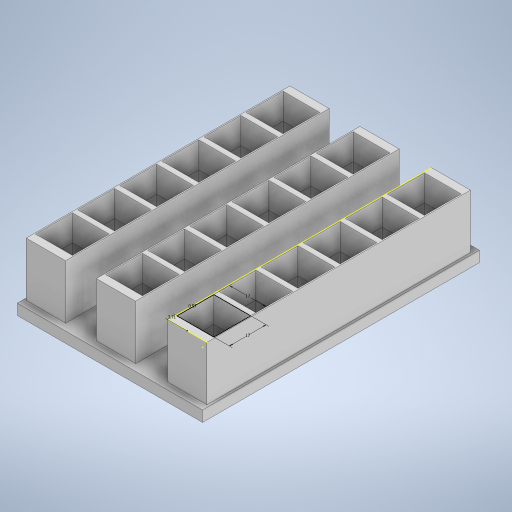
# Autodesk Inventor part: cuvettestorage3_6x3
Saved by Autodesk Inventor 2023 (Build 270158000, 158)
## iProperties
Created: 2024-07-02
Part Number: cuvettestorage3_6x3
Material: Generic
Document SubType Name: Modeling
Designer: storm
Density: 1 g/cm^3
Appearance: Default
Author: storm
Autodesk Inventor part; units mm, degrees
ref_plane "YZ Plane" through (0, 0, 0) normal (1, 0, 0) x (0, 1, 0)
ref_plane "XZ Plane" through (0, 0, 0) normal (0, 1, 0) x (-1, 0, 0)
ref_plane "XY Plane" through (0, 0, 0) normal (0, 0, 1) x (1, 0, 0)
sketch "Sketch1" plane through (0, 0, 0) normal (0, 1, 0) x (-1, 0, 0)
  line L0 (0, 0) -> (85.5, 0)
  line L1 (85.5, 0) -> (85.5, -127.8)
  line L2 (85.5, -127.8) -> (0, -127.8)
  line L3 (0, -127.8) -> (0, 0)
  dimension "d0" = 127.8
  dimension "d1" = 85.5
  constraints: 8 end point, 2 parallel, 1 horizontal, 1 perpendicular
  measures "d0" distance of L0.end L1.end
  measures "d1" distance between parallel lines of L3 L1
extrude "Extrusion1" add sketch "Sketch1" along normal blind 5
sketch "Sketch2" plane through (0, 5, 0) normal (0, 1, 0) x (1, 0, 0)
  line L0 (-84.43, 3.05) -> (-66.3, 3.05)
  line L1 (-66.3, 3.05) -> (-66.3, 124.74)
  line L2 (-66.3, 124.74) -> (-84.43, 124.74)
  line L3 (-84.43, 124.74) -> (-84.43, 3.05)
  line L4 (-52.08, 3.05) -> (-33.95, 3.05)
  line L5 (-33.95, 3.05) -> (-33.95, 124.74)
  line L6 (-33.95, 124.74) -> (-52.08, 124.74)
  line L7 (-52.08, 124.74) -> (-52.08, 3.05)
  line L8 (-19.18, 3.05) -> (-1.05, 3.05)
  line L9 (-1.05, 3.05) -> (-1.05, 124.74)
  line L10 (-1.05, 124.74) -> (-19.18, 124.74)
  line L11 (-19.18, 124.74) -> (-19.18, 3.05)
  line L12 (0, 0) -> (0, 127.8) projected
  line L13 (-85.5, 0) -> (0, 0) projected
  point P0 (-10.115, 124.74)
  point P1 (-10.115, 3.05)
  dimension "d4" = 18.13
  dimension "d5" = 121.69
  dimension "d6" = 1.05
  dimension "d7" = 3.05
  dimension "d8" = 14.77
  dimension "d9" = 18.13
  dimension "d10" = 14.22
  dimension "d11" = 18.13
  constraints: 24 end point, 6 parallel, 4 point on line, 3 horizontal, 3 perpendicular, 2 midpoint
  measures "d4" distance between parallel lines of L9 L11
  measures "d5" distance of point (-10.115, 124.74) point (-10.115, 3.05)
  measures "d6" distance between parallel lines of L12 L9
  measures "d7" distance between parallel lines of L13 L8
  measures "d8" distance between parallel lines of L11 L5
  measures "d9" distance between parallel lines of L5 L7
  measures "d10" distance between parallel lines of L7 L1
  measures "d11" distance between parallel lines of L1 L3
extrude "Extrusion2" add sketch "Sketch2" along normal blind 25
sketch "Sketch3" plane through (0, 30, 0) normal (0, 1, 0) x (1, 0, 0)
  line L0 (-19.18, 124.74) -> (-19.18, 3.05) projected
  line L1 (-1.05, 3.05) -> (-1.05, 124.74) projected
  line L2 (-19.18, 3.05) -> (-1.05, 3.05) projected
  line L3 (-16.615, 28.214) -> (-3.615, 28.214)
  line L4 (-3.615, 28.214) -> (-3.615, 41.214)
  line L5 (-3.615, 41.214) -> (-16.615, 41.214)
  line L6 (-16.615, 41.214) -> (-16.615, 28.214)
  line L7 (-16.615, 47.668) -> (-3.615, 47.668)
  line L8 (-3.615, 47.668) -> (-3.615, 60.668)
  line L9 (-3.615, 60.668) -> (-16.615, 60.668)
  line L10 (-16.615, 60.668) -> (-16.615, 47.668)
  line L11 (-16.615, 67.122) -> (-3.615, 67.122)
  line L12 (-3.615, 67.122) -> (-3.615, 80.122)
  line L13 (-3.615, 80.122) -> (-16.615, 80.122)
  line L14 (-16.615, 80.122) -> (-16.615, 67.122)
  line L15 (-16.615, 86.576) -> (-3.615, 86.576)
  line L16 (-3.615, 86.576) -> (-3.615, 99.576)
  line L17 (-3.615, 99.576) -> (-16.615, 99.576)
  line L18 (-16.615, 99.576) -> (-16.615, 86.576)
  line L19 (-16.615, 106.03) -> (-3.615, 106.03)
  line L20 (-3.615, 106.03) -> (-3.615, 119.03)
  line L21 (-3.615, 119.03) -> (-16.615, 119.03)
  line L22 (-16.615, 119.03) -> (-16.615, 106.03)
  line L23 (-1.05, 124.74) -> (-19.18, 124.74) projected
  line L24 (-52.08, 124.74) -> (-52.08, 3.05) projected
  line L25 (-33.95, 3.05) -> (-33.95, 124.74) projected
  line L26 (-52.08, 3.05) -> (-33.95, 3.05) projected
  line L27 (-84.43, 124.74) -> (-84.43, 3.05) projected
  line L28 (-66.3, 3.05) -> (-66.3, 124.74) projected
  line L29 (-84.43, 3.05) -> (-66.3, 3.05) projected
  line L30 (-16.615, 8.76) -> (-3.615, 8.76)
  line L31 (-3.615, 8.76) -> (-3.615, 21.76)
  line L32 (-3.615, 21.76) -> (-16.615, 21.76)
  line L33 (-16.615, 21.76) -> (-16.615, 8.76)
  line L34 (-33.95, 124.74) -> (-52.08, 124.74) projected
  line L35 (-49.515, 8.76) -> (-36.515, 8.76)
  line L36 (-36.515, 8.76) -> (-36.515, 21.76)
  line L37 (-36.515, 21.76) -> (-49.515, 21.76)
  line L38 (-49.515, 21.76) -> (-49.515, 8.76)
  line L39 (-49.515, 28.214) -> (-36.515, 28.214)
  line L40 (-36.515, 28.214) -> (-36.515, 41.214)
  line L41 (-36.515, 41.214) -> (-49.515, 41.214)
  line L42 (-49.515, 41.214) -> (-49.515, 28.214)
  line L43 (-49.515, 47.668) -> (-36.515, 47.668)
  line L44 (-36.515, 47.668) -> (-36.515, 60.668)
  line L45 (-36.515, 60.668) -> (-49.515, 60.668)
  line L46 (-49.515, 60.668) -> (-49.515, 47.668)
  line L47 (-49.515, 67.122) -> (-36.515, 67.122)
  line L48 (-36.515, 67.122) -> (-36.515, 80.122)
  line L49 (-36.515, 80.122) -> (-49.515, 80.122)
  line L50 (-49.515, 80.122) -> (-49.515, 67.122)
  line L51 (-49.515, 86.576) -> (-36.515, 86.576)
  line L52 (-36.515, 86.576) -> (-36.515, 99.576)
  line L53 (-36.515, 99.576) -> (-49.515, 99.576)
  line L54 (-49.515, 99.576) -> (-49.515, 86.576)
  line L55 (-49.515, 106.03) -> (-36.515, 106.03)
  line L56 (-36.515, 106.03) -> (-36.515, 119.03)
  line L57 (-36.515, 119.03) -> (-49.515, 119.03)
  line L58 (-49.515, 119.03) -> (-49.515, 106.03)
  line L59 (-81.865, 8.76) -> (-68.865, 8.76)
  line L60 (-68.865, 8.76) -> (-68.865, 21.76)
  line L61 (-68.865, 21.76) -> (-81.865, 21.76)
  line L62 (-81.865, 21.76) -> (-81.865, 8.76)
  line L63 (-81.865, 28.214) -> (-68.865, 28.214)
  line L64 (-68.865, 28.214) -> (-68.865, 41.214)
  line L65 (-68.865, 41.214) -> (-81.865, 41.214)
  line L66 (-81.865, 41.214) -> (-81.865, 28.214)
  line L67 (-81.865, 47.668) -> (-68.865, 47.668)
  line L68 (-68.865, 47.668) -> (-68.865, 60.668)
  line L69 (-68.865, 60.668) -> (-81.865, 60.668)
  line L70 (-81.865, 60.668) -> (-81.865, 47.668)
  line L71 (-81.865, 67.122) -> (-68.865, 67.122)
  line L72 (-68.865, 67.122) -> (-68.865, 80.122)
  line L73 (-68.865, 80.122) -> (-81.865, 80.122)
  line L74 (-81.865, 80.122) -> (-81.865, 67.122)
  line L75 (-81.865, 86.576) -> (-68.865, 86.576)
  line L76 (-68.865, 86.576) -> (-68.865, 99.576)
  line L77 (-68.865, 99.576) -> (-81.865, 99.576)
  line L78 (-81.865, 99.576) -> (-81.865, 86.576)
  line L79 (-81.865, 106.03) -> (-68.865, 106.03)
  line L80 (-68.865, 106.03) -> (-68.865, 119.03)
  line L81 (-68.865, 119.03) -> (-81.865, 119.03)
  line L82 (-81.865, 119.03) -> (-81.865, 106.03)
  line L83 (-66.3, 124.74) -> (-84.43, 124.74) projected
  point P0 (0, 0)
  point P1 (-16.615, 13.26)
  point P2 (-3.615, 13.26)
  point P3 (-10.115, 60.668)
  point P4 (-10.115, 47.668)
  point P5 (-3.615, 54.168)
  point P6 (-16.615, 54.168)
  point P7 (-16.615, 73.622)
  point P8 (-3.615, 93.076)
  point P9 (-16.615, 93.076)
  point P10 (-3.615, 112.53)
  point P11 (-16.615, 112.53)
  point P12 (-3.615, 34.714)
  point P13 (-1.05, 63.895)
  point P14 (-10.115, 80.122)
  point P15 (-10.115, 41.214)
  point P16 (-10.115, 28.214)
  point P17 (-43.015, 3.05)
  point P18 (-75.365, 3.05)
  point P19 (-10.115, 8.76)
  point P20 (-10.115, 3.05)
  point P21 (-43.015, 124.74)
  point P22 (-43.015, 8.76)
  point P23 (-49.515, 15.26)
  point P24 (-75.365, 21.76)
  point P25 (-75.365, 67.122)
  point P26 (-75.365, 60.668)
  point P27 (-75.365, 106.03)
  point P28 (-75.365, 99.576)
  point P29 (-75.365, 124.74)
  point P30 (-68.865, 15.26)
  dimension "d19" = 13
  dimension "d20" = 13
  dimension "d21" = 13
  dimension "d22" = 13
  dimension "d23" = 13
  dimension "d24" = 13
  dimension "d25" = 13
  dimension "d26" = 13
  dimension "d27" = 13
  dimension "d28" = 13
  dimension "d29" = 5.71
  dimension "d33" = 2.565
  dimension "d34" = 2.565
  dimension "d35" = 2.565
  dimension "d36" = 2.565
  dimension "d37" = 2.565
  dimension "d38" = 2.565
  dimension "d39" = 2.565
  dimension "d40" = 121.69
  dimension "d41" = 6.454
  dimension "d42" = 6.454
  dimension "d43" = 6.454
  dimension "d44" = 6.454
  dimension "d67" = 6.454
  dimension "d68" = 5.71
  dimension "d78" = 13
  dimension "d79" = 13
  dimension "d80" = 5.71
  dimension "d81" = 2.565
  dimension "d82" = 2.565
  dimension "d83" = 6.454
  dimension "d84" = 6.454
  dimension "d85" = 6.454
  dimension "d86" = 6.454
  dimension "d87" = 6.454
  dimension "d88" = 13
  dimension "d89" = 5.71
  dimension "d90" = 6.454
  dimension "d91" = 6.454
  dimension "d92" = 6.454
  dimension "d93" = 6.454
  dimension "d94" = 6.454
  dimension "d95" = 5.71
  dimension "d96" = 2.565
  constraints: 144 end point, 36 parallel, 28 midpoint, 24 point on line, 18 horizontal, 18 perpendicular
  measures "d19" distance of L4.end L3.end
  measures "d20" distance between parallel lines of L4 L6
  measures "d21" distance of point (-10.115, 60.668) point (-10.115, 47.668)
  measures "d22" distance of point (-3.615, 54.168) point (-16.615, 54.168)
  measures "d23" distance from line of L12 point (-16.615, 73.622)
  measures "d24" distance between parallel lines of L13 L11
  measures "d25" distance of point (-3.615, 93.076) point (-16.615, 93.076)
  measures "d26" distance between parallel lines of L17 L15
  measures "d27" distance of point (-3.615, 112.53) point (-16.615, 112.53)
  measures "d28" distance between parallel lines of L21 L19
  measures "d29" distance between parallel lines of L23 L21
  measures "d33" distance between parallel lines of L0 L6
  measures "d34" distance from line of L1 point (-3.615, 34.714)
  measures "d35" distance between parallel lines of L0 L10
  measures "d36" distance between parallel lines of L0 L14
  measures "d37" distance from line of point (-1.05, 63.895) L12
  measures "d38" distance between parallel lines of L0 L18
  measures "d39" distance between parallel lines of L0 L22
  measures "d40" distance between parallel lines of L23 L2
  measures "d41" distance between parallel lines of L19 L17
  measures "d42" distance from line of point (-10.115, 80.122) L15
  measures "d43" distance between parallel lines of L9 L11
  measures "d44" distance from line of point (-10.115, 41.214) L7
  measures "d67" distance between parallel lines of L3 L32
  measures "d68" distance of point (-10.115, 8.76) point (-10.115, 3.05)
  measures "d78" distance of L37.end L36.end
  measures "d79" distance of L36.end L35.end
  measures "d80" distance from line of L26 point (-43.015, 8.76)
  measures "d81" distance between parallel lines of L25 L36
  measures "d82" distance from line of L24 point (-49.515, 15.26)
  measures "d83" distance between parallel lines of L39 L37
  measures "d84" distance between parallel lines of L43 L41
  measures "d85" distance between parallel lines of L47 L45
  measures "d86" distance between parallel lines of L51 L49
  measures "d87" distance between parallel lines of L55 L53
  measures "d88" distance of L61.end L60.end
  measures "d89" distance between parallel lines of L59 L29
  measures "d90" distance from line of L63 point (-75.365, 21.76)
  measures "d91" distance between parallel lines of L67 L65
  measures "d92" distance of point (-75.365, 67.122) point (-75.365, 60.668)
  measures "d93" distance between parallel lines of L75 L73
  measures "d94" distance of point (-75.365, 106.03) point (-75.365, 99.576)
  measures "d95" distance from line of L81 point (-75.365, 124.74)
  measures "d96" distance from line of L28 point (-68.865, 15.26)
extrude "Extrusion3" cut sketch "Sketch3" against normal blind 20 contours L6 L5 L4 L3 | L10 L9 L8 L7 | L14 L13 L12 L11 | L18 L17 L16 L15 | L22 L21 L20 L19
sketch "Sketch4" plane through (0, 30, 0) normal (0, 1, 0) x (1, 0, 0)
  line L0 (-16.615, 21.76) -> (-3.615, 21.76)
  line L1 (-3.615, 21.76) -> (-3.615, 8.76)
  line L2 (-3.615, 8.76) -> (-16.615, 8.76)
  line L3 (-16.615, 8.76) -> (-16.615, 21.76)
  line L4 (-19.18, 124.74) -> (-19.18, 3.05) projected
  line L5 (-1.05, 3.05) -> (-1.05, 124.74) projected
  line L6 (-19.18, 3.05) -> (-1.05, 3.05) projected
  point P0 (0, 0)
  point P1 (-16.615, 15.26)
  point P2 (-3.615, 15.26)
  point P3 (-10.115, 3.05)
  point P4 (-10.115, 8.76)
  dimension "d56" = 13
  dimension "d57" = 13
  dimension "d58" = 2.565
  dimension "d59" = 2.565
  dimension "d60" = 5.71
  constraints: 8 end point, 4 midpoint, 2 parallel, 1 horizontal, 1 perpendicular
  measures "d56" distance of L1.end L2.end
  measures "d57" distance of L0.end L1.end
  measures "d58" distance from line of L4 point (-16.615, 15.26)
  measures "d59" distance from line of L5 point (-3.615, 15.26)
  measures "d60" distance of point (-10.115, 3.05) point (-10.115, 8.76)
extrude "Extrusion4" cut sketch "Sketch4" against normal blind 20
sketch "Sketch5" plane through (0, 30, 0) normal (0, 1, 0) x (1, 0, 0)
  line L0 (-18.61, 6.76) -> (-1.61, 6.76)
  line L1 (-1.61, 6.76) -> (-1.61, 23.76)
  line L2 (-1.61, 23.76) -> (-18.61, 23.76)
  line L3 (-18.61, 23.76) -> (-18.61, 6.76)
  line L4 (-19.18, 124.74) -> (-19.18, 3.05) projected
  line L5 (-19.18, 3.05) -> (-1.05, 3.05) projected
  point P0 (0, 0)
  point P1 (-10.115, 3.05)
  dimension "d63" = 17
  dimension "d64" = 17
  dimension "d65" = 0.57
  dimension "d66" = 3.71
  constraints: 8 end point, 2 parallel, 1 horizontal, 1 midpoint, 1 perpendicular
  measures "d63" distance of L2.end L1.end
  measures "d64" distance of L1.end L0.end
  measures "d65" distance between parallel lines of L3 L4
  measures "d66" distance from line of point (-10.115, 3.05) L0
chamfer "Chamfer6" distance 2 distance2 10 24 edges at (-10.115, 30, -8.76) (-16.615, 30, -15.26) (-3.615, 30, -15.26) (-10.115, 30, -21.76) (-16.615, 30, -34.714) (-10.115, 30, -28.214) (-10.115, 30, -41.214) (-3.615, 30, -34.714) (-3.615, 30, -54.168) (-10.115, 30, -47.668) (-16.615, 30, -54.168) (-10.115, 30, -60.668) (-16.615, 30, -73.622) (-10.115, 30, -67.122) (-3.615, 30, -73.622) (-10.115, 30, -80.122) (-10.115, 30, -86.576) (-16.615, 30, -93.076) (-3.615, 30, -93.076) (-10.115, 30, -99.576) (-10.115, 30, -106.03) (-16.615, 30, -112.53) (-10.115, 30, -119.03) (-3.615, 30, -112.53) measured on face at (-1.905, 30, -56.3347)
sketch "Sketch6" plane through (0, 30, 0) normal (0, 1, 0) x (1, 0, 0)
  line L0 (-49.515, 8.76) -> (-36.515, 8.76)
  line L1 (-36.515, 8.76) -> (-36.515, 21.76)
  line L2 (-36.515, 21.76) -> (-49.515, 21.76)
  line L3 (-49.515, 21.76) -> (-49.515, 8.76)
  line L4 (-52.08, 124.74) -> (-52.08, 3.05) projected
  line L5 (-52.08, 3.05) -> (-33.95, 3.05) projected
  line L6 (-33.95, 3.05) -> (-33.95, 124.74) projected
  line L7 (-36.515, 28.214) -> (-49.515, 28.214)
  line L8 (-49.515, 28.214) -> (-49.515, 41.214)
  line L9 (-49.515, 41.214) -> (-36.515, 41.214)
  line L10 (-36.515, 41.214) -> (-36.515, 28.214)
  line L11 (-36.515, 47.668) -> (-49.515, 47.668)
  line L12 (-49.515, 47.668) -> (-49.515, 60.668)
  line L13 (-49.515, 60.668) -> (-36.515, 60.668)
  line L14 (-36.515, 60.668) -> (-36.515, 47.668)
  line L15 (-36.515, 67.122) -> (-49.515, 67.122)
  line L16 (-49.515, 67.122) -> (-49.515, 80.122)
  line L17 (-49.515, 80.122) -> (-36.515, 80.122)
  line L18 (-36.515, 80.122) -> (-36.515, 67.122)
  line L19 (-36.515, 86.576) -> (-49.515, 86.576)
  line L20 (-49.515, 86.576) -> (-49.515, 99.576)
  line L21 (-49.515, 99.576) -> (-36.515, 99.576)
  line L22 (-36.515, 99.576) -> (-36.515, 86.576)
  line L23 (-36.515, 106.03) -> (-49.515, 106.03)
  line L24 (-49.515, 106.03) -> (-49.515, 119.03)
  line L25 (-49.515, 119.03) -> (-36.515, 119.03)
  line L26 (-36.515, 119.03) -> (-36.515, 106.03)
  line L27 (-33.95, 124.74) -> (-52.08, 124.74) projected
  line L28 (-3.615, 28.214) -> (-16.615, 28.214) projected
  line L29 (-16.615, 21.76) -> (-3.615, 21.76) projected
  point P0 (0, 0)
  point P1 (-49.515, 15.26)
  point P2 (-43.015, 3.05)
  point P3 (-43.015, 8.76)
  point P4 (-43.015, 119.03)
  dimension "d115" = 13
  dimension "d116" = 13
  dimension "d117" = 2.565
  dimension "d118" = 5.71
  dimension "d119" = 2.565
  dimension "d120" = 13
  dimension "d121" = 13
  dimension "d122" = 13
  dimension "d123" = 13
  dimension "d124" = 13
  dimension "d125" = 13
  dimension "d126" = 13
  dimension "d127" = 5.71
  dimension "d128" = 6.454
  dimension "d129" = 6.454
  dimension "d130" = 6.454
  dimension "d131" = 6.454
  dimension "d132" = 6.454
  dimension "d133" = 6.454
  constraints: 48 end point, 12 parallel, 7 point on line, 6 horizontal, 6 perpendicular, 4 midpoint
  measures "d115" distance of L2.end L1.end
  measures "d116" distance of L1.end L0.end
  measures "d117" distance from line of L4 point (-49.515, 15.26)
  measures "d118" distance of point (-43.015, 3.05) point (-43.015, 8.76)
  measures "d119" distance between parallel lines of L6 L1
  measures "d120" distance of L8.end L9.end
  measures "d121" distance of L7.end L8.end
  measures "d122" distance of L12.end L13.end
  measures "d123" distance of L11.end L12.end
  measures "d124" distance of L15.end L16.end
  measures "d125" distance of L19.end L20.end
  measures "d126" distance of L23.end L24.end
  measures "d127" distance from line of L27 point (-43.015, 119.03)
  measures "d128" distance between parallel lines of L28 L29
  measures "d129" distance between parallel lines of L7 L2
  measures "d130" distance between parallel lines of L11 L9
  measures "d131" distance between parallel lines of L15 L13
  measures "d132" distance between parallel lines of L19 L17
  measures "d133" distance between parallel lines of L23 L21
extrude "Extrusion5" cut sketch "Sketch6" against normal blind 20 contours L3 L2 L1 L0 | L7 L8 L9 L10 | L11 L12 L13 L14 | L15 L16 L17 L18 | L19 L20 L21 L22 | L23 L24 L25 L26
chamfer "Chamfer7" distance 2 distance2 10 24 edges at (-43.015, 30, -8.76) (-49.515, 30, -15.26) (-43.015, 30, -21.76) (-36.515, 30, -15.26) (-43.015, 30, -28.214) (-49.515, 30, -34.714) (-43.015, 30, -41.214) (-36.515, 30, -34.714) (-43.015, 30, -47.668) (-49.515, 30, -54.168) (-43.015, 30, -60.668) (-36.515, 30, -54.168) (-43.015, 30, -67.122) (-49.515, 30, -73.622) (-43.015, 30, -80.122) (-36.515, 30, -73.622) (-43.015, 30, -86.576) (-49.515, 30, -93.076) (-43.015, 30, -99.576) (-36.515, 30, -93.076) (-43.015, 30, -106.03) (-49.515, 30, -112.53) (-43.015, 30, -119.03) (-36.515, 30, -112.53) measured on face at (-51.225, 30, -49.85)
sketch "Sketch7" plane through (0, 30, 0) normal (0, 1, 0) x (1, 0, 0)
  line L0 (-81.865, 8.76) -> (-68.865, 8.76)
  line L1 (-68.865, 8.76) -> (-68.865, 21.76)
  line L2 (-68.865, 21.76) -> (-81.865, 21.76)
  line L3 (-81.865, 21.76) -> (-81.865, 8.76)
  line L4 (-84.43, 124.74) -> (-84.43, 3.05) projected
  line L5 (-66.3, 3.05) -> (-66.3, 124.74) projected
  line L6 (-84.43, 3.05) -> (-66.3, 3.05) projected
  line L7 (-81.865, 28.214) -> (-68.865, 28.214)
  line L8 (-68.865, 28.214) -> (-68.865, 41.214)
  line L9 (-68.865, 41.214) -> (-81.865, 41.214)
  line L10 (-81.865, 41.214) -> (-81.865, 28.214)
  line L11 (-81.865, 47.668) -> (-68.865, 47.668)
  line L12 (-68.865, 47.668) -> (-68.865, 60.668)
  line L13 (-68.865, 60.668) -> (-81.865, 60.668)
  line L14 (-81.865, 60.668) -> (-81.865, 47.668)
  line L15 (-81.865, 67.122) -> (-68.865, 67.122)
  line L16 (-68.865, 67.122) -> (-68.865, 80.122)
  line L17 (-68.865, 80.122) -> (-81.865, 80.122)
  line L18 (-81.865, 80.122) -> (-81.865, 67.122)
  line L19 (-81.865, 86.576) -> (-68.865, 86.576)
  line L20 (-68.865, 86.576) -> (-68.865, 99.576)
  line L21 (-68.865, 99.576) -> (-81.865, 99.576)
  line L22 (-81.865, 99.576) -> (-81.865, 86.576)
  line L23 (-81.865, 106.03) -> (-68.865, 106.03)
  line L24 (-68.865, 106.03) -> (-68.865, 119.03)
  line L25 (-68.865, 119.03) -> (-81.865, 119.03)
  line L26 (-81.865, 119.03) -> (-81.865, 106.03)
  line L27 (-66.3, 124.74) -> (-84.43, 124.74) projected
  line L28 (-36.515, 67.122) -> (-49.515, 67.122) projected
  line L29 (-49.515, 60.668) -> (-36.515, 60.668) projected
  point P0 (0, 0)
  point P1 (-75.365, 3.05)
  point P2 (-75.365, 8.76)
  point P3 (-75.365, 124.74)
  point P4 (-75.365, 99.576)
  point P5 (-75.365, 86.576)
  point P6 (-75.365, 47.668)
  dimension "d139" = 13
  dimension "d140" = 13
  dimension "d141" = 2.565
  dimension "d142" = 2.565
  dimension "d143" = 5.71
  dimension "d144" = 13
  dimension "d145" = 13
  dimension "d146" = 13
  dimension "d147" = 13
  dimension "d148" = 13
  dimension "d149" = 13
  dimension "d150" = 5.71
  dimension "d151" = 6.454
  dimension "d152" = 6.454
  dimension "d153" = 6.454
  dimension "d154" = 6.454
  dimension "d155" = 6.454
  dimension "d156" = 6.454
  constraints: 48 end point, 12 parallel, 8 point on line, 6 horizontal, 6 midpoint, 6 perpendicular
  measures "d139" distance of L2.end L1.end
  measures "d140" distance of L1.end L0.end
  measures "d141" distance between parallel lines of L4 L3
  measures "d142" distance between parallel lines of L5 L1
  measures "d143" distance of point (-75.365, 3.05) point (-75.365, 8.76)
  measures "d144" distance of L9.end L8.end
  measures "d145" distance of L8.end L7.end
  measures "d146" distance of L12.end L11.end
  measures "d147" distance of L16.end L15.end
  measures "d148" distance of L20.end L19.end
  measures "d149" distance of L24.end L23.end
  measures "d150" distance from line of point (-75.365, 124.74) L25
  measures "d151" distance between parallel lines of L28 L29
  measures "d152" distance from line of L23 point (-75.365, 99.576)
  measures "d153" distance from line of L17 point (-75.365, 86.576)
  measures "d154" distance between parallel lines of L13 L15
  measures "d155" distance from line of L9 point (-75.365, 47.668)
  measures "d156" distance between parallel lines of L2 L7
extrude "Extrusion6" cut sketch "Sketch7" against normal blind 20 contours L3 L2 L1 L0 | L10 L9 L8 L7 | L14 L13 L12 L11 | L18 L17 L16 L15 | L22 L21 L20 L19 | L26 L25 L24 L23
chamfer "Chamfer8" distance 2 distance2 10 24 edges at (-81.865, 30, -15.26) (-75.365, 30, -8.76) (-68.865, 30, -15.26) (-75.365, 30, -21.76) (-75.365, 30, -28.214) (-81.865, 30, -34.714) (-75.365, 30, -41.214) (-68.865, 30, -34.714) (-75.365, 30, -47.668) (-81.865, 30, -54.168) (-75.365, 30, -60.668) (-68.865, 30, -54.168) (-75.365, 30, -67.122) (-81.865, 30, -73.622) (-75.365, 30, -80.122) (-68.865, 30, -73.622) (-75.365, 30, -86.576) (-81.865, 30, -93.076) (-75.365, 30, -99.576) (-68.865, 30, -93.076) (-68.865, 30, -112.53) (-75.365, 30, -106.03) (-81.865, 30, -112.53) (-75.365, 30, -119.03) measured on face at (-83.575, 30, -75.7887)
body "Solid1"
